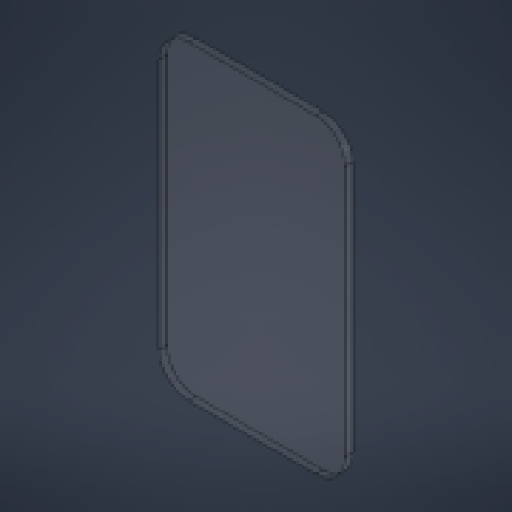
# Autodesk Inventor part: Door Panel Front Panel
Saved by Autodesk Inventor 2026 (Build 300175050, 175E)
## iProperties
Created: 2025-05-22
Part Number: Door Panel Front Panel
Material: Polycarbonate, Clear
Document SubType Name: Modeling
Designer: Joshua Eah
Density: 1.2 g/cm^3
Appearance: Polycarbonate - Clear
Author: Joshua Eah
Autodesk Inventor part; units mm, degrees
ref_plane "YZ Plane" through (0, 0, 0) normal (1, 0, 0) x (0, 1, 0)
ref_plane "XZ Plane" through (0, 0, 0) normal (0, 1, 0) x (-1, 0, 0)
ref_plane "XY Plane" through (0, 0, 0) normal (0, 0, 1) x (1, 0, 0)
sketch "Sketch1" plane through (0, 0, 0) normal (0, 0, 1) x (1, 0, 0)
  line L0 (0, 0) -> (159.8, 0)
  line L1 (159.8, 0) -> (159.8, 267.15)
  line L2 (159.8, 267.15) -> (0, 267.15)
  line L3 (0, 267.15) -> (0, 0)
  dimension "d0" = 159.8
  dimension "d1" = 267.15
  constraints: 8 end point, 2 parallel, 1 horizontal, 1 perpendicular
  measures "d0" distance of L2.end L1.end
  measures "d1" distance of L1.end L0.end
extrude "Extrusion1" add sketch "Sketch1" along normal blind 6.35
fillet "Fillet1" radius 25.4 4 edges at (159.8, 0, 3.175) (0, 0, 3.175) (0, 267.15, 3.175) (159.8, 267.15, 3.175)
body "Solid1"
